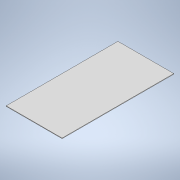
# Autodesk Inventor part: back
Saved by Autodesk Inventor 2021 (Build 250183000, 183)
## iProperties
Created: 2021-03-25
Part Number: back
Material: Generic
Document SubType Name: Modeling
Designer: noori
Density: 1 g/cm^3
Appearance: Default
Author: noori
Autodesk Inventor part; units mm, degrees
ref_plane "YZ Plane" through (0, 0, 0) normal (1, 0, 0) x (0, 1, 0)
ref_plane "XZ Plane" through (0, 0, 0) normal (0, 1, 0) x (-1, 0, 0)
ref_plane "XY Plane" through (0, 0, 0) normal (0, 0, 1) x (1, 0, 0)
sketch "Sketch1" plane through (0, 0, 0) normal (0, 1, 0) x (-1, 0, 0)
  line L0 (200, 400) -> (-200, 400)
  line L1 (-200, 400) -> (-200, -400)
  line L2 (-200, -400) -> (200, -400)
  line L3 (200, -400) -> (200, 400)
  point P0 (0, 0)
  dimension "d0" = 800
  dimension "d1" = 400
  dimension "d2" = 200
  dimension "d3" = 400
  constraints: 8 end point, 2 parallel, 1 horizontal, 1 perpendicular
  measures "d0" distance of L2.end L0.start
  measures "d1" distance of L1.end L2.end
  measures "d2" distance from line of L3 point (0, 0)
  measures "d3" distance from line of L0 point (0, 0)
extrude "Extrusion1" add sketch "Sketch1" along normal blind 4
body "Solid1"
